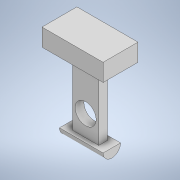
# Autodesk Inventor part: Example Follower
Saved by Autodesk Inventor 2021 (Build 250183000, 183)
## iProperties
Created: 2021-03-09
Part Number: Example Follower
Material: Generic
Document SubType Name: Modeling
Designer: Jawal
Density: 1 g/cm^3
Appearance: Default
Author: Jawal
Autodesk Inventor part; units mm, degrees
ref_plane "YZ Plane" through (0, 0, 0) normal (1, 0, 0) x (0, 1, 0)
ref_plane "XZ Plane" through (0, 0, 0) normal (0, 1, 0) x (-1, 0, 0)
ref_plane "XY Plane" through (0, 0, 0) normal (0, 0, 1) x (1, 0, 0)
sketch "Sketch1" plane through (0, 0, 0) normal (1, 0, 0) x (0, 1, 0)
  line L0 (50, 10) -> (40, 10)
  line L1 (40, 10) -> (40, -10)
  line L2 (40, -10) -> (50, -10)
  line L3 (50, -10) -> (50, 10)
  line L4 (40, 2.5) -> (0, 2.5)
  line L5 (0, 2.5) -> (0, -2.5)
  line L6 (0, -2.5) -> (40, -2.5)
  line L7 (40, -2.5) -> (40, 2.5)
  point P0 (0, 0)
  dimension "d0" = 40
  dimension "d1" = 10
  dimension "d2" = 5
  dimension "d3" = 2.5
  dimension "d4" = 20
  dimension "d5" = 10
  constraints: 16 end point, 4 parallel, 2 horizontal, 2 perpendicular, 1 point on line
  measures "d0" distance of L5.end L6.end
  measures "d1" distance of L1.end L2.end
  measures "d2" distance of L4.end L5.end
  measures "d3" distance from line of L6 point (0, 0)
  measures "d4" distance of L2.end L0.start
  measures "d5" distance from line of point (0, 0) L2
extrude "Extrusion1" add sketch "Sketch1" along normal blind 15
sketch "Sketch2" plane through (15, 0, 0) normal (1, 0, 0) x (0, 0, -1)
  line L0 (-10, 50) -> (-10, 40) projected
  line L1 (2.5, 40) -> (10, 40) projected
  line L2 (-10, 50) -> (10, 50)
  line L3 (10, 50) -> (10, 40)
  line L4 (10, 40) -> (-10, 40)
  line L5 (-10, 40) -> (-10, 50)
  point P0 (0, 0)
  constraints: 8 end point, 2 parallel, 1 horizontal, 1 perpendicular
extrude "Extrusion2" add sketch "Sketch2" along normal blind 10
sketch "Sketch3" plane through (0, 0, 0) normal (-1, 0, 0) x (0, 0, 1)
  line L0 (-10, 40) -> (-10, 50) projected
  line L1 (10, 50) -> (10, 40) projected
  line L2 (-10, 50) -> (10, 50)
  line L3 (10, 50) -> (10, 40)
  line L4 (10, 40) -> (-10, 40)
  line L5 (-10, 40) -> (-10, 50)
  point P0 (0, 0)
  constraints: 8 end point, 2 parallel, 1 horizontal, 1 perpendicular
extrude "Extrusion3" add sketch "Sketch3" along normal blind 10
sketch "Sketch4" plane through (0, 0, -2.5) normal (0, 0, -1) x (-1, 0, 0)
  circle A0 centre (-7.5, 12) radius 6
  point P0 (0, 0)
  dimension "d12" = 12
  constraints: 1 centre point
  measures "d12" diameter of A0
extrude "Extrusion4" cut sketch "Sketch4" against normal blind 5
sketch "Sketch5" plane through (0, 0, -2.5) normal (0, -1, 0) x (1, 0, 0)
  line L0 (-5, 7.5) -> (20, 7.5)
  line L1 (20, 7.5) -> (20, -2.5)
  line L2 (20, -2.5) -> (-5, -2.5)
  line L3 (-5, -2.5) -> (-5, 7.5)
  point P0 (0, 2.5)
  dimension "d15" = 25
  dimension "d16" = 10
  constraints: 8 end point, 2 parallel, 1 horizontal, 1 perpendicular
  measures "d15" distance of L1.end L2.end
  measures "d16" distance of L0.end L1.end
extrude "Extrusion5" add sketch "Sketch5" along normal blind 10
sketch "Sketch6" plane through (20, 0, 5) normal (1, 0, 0) x (0, 0, -1)
  line L0 (0, 0) -> (10, 0) projected
  arc A0 (0, 0) -> (10, 0) centre (5, 0) ccw
  line L1 (0, 0) -> (0, -10) projected
  line L2 (0, 0) -> (0, -10)
  line L3 (10, -10) -> (0, -10) projected
  line L4 (0, -10) -> (10, -10)
  line L5 (10, 0) -> (10, -10) projected
  line L6 (10, -10) -> (10, 0)
  point P0 (5, 0)
  dimension "d19" = 5
  constraints: 6 end point, 2 collinear, 2 point on circle, 1 centre point, 1 perpendicular
  measures "d19" radius of A0
extrude "Extrusion6" cut sketch "Sketch6" against normal blind 25 contours A0 L5 L3 L1
equation "\"d3\" = 0.5 * d2"
equation "\"d5\" = 0.5 * d4"
body "Solid1"
